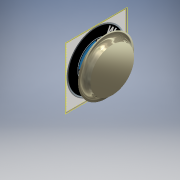
# Autodesk Inventor part: BMW Cap dish decal ready to attach
Saved by Autodesk Inventor 2016 (Build 200138000, 138)
## iProperties
Created: 2016-02-13
Part Number: BMW Cap dish decal ready to attach
Material: Brass, Soft Yellow
Document SubType Name: Modeling
Designer: Amilod
Density: 8.47 g/cm^3
Appearance: Nickel
Mass: 13200.3 g
Surface Area: 11659.4 cm^2
Volume: 4888.99 cm^3
Author: Amilod
Autodesk Inventor part; units mm, degrees
ref_plane "XZ Plane" through (0, 0, 0) normal (0, 1, 0) x (-1, 0, 0)
ref_plane "XY Plane" through (0, 0, 0) normal (0, 0, 1) x (1, 0, 0)
ref_plane "Work Plane5" through (-81, 0, 0) normal (1, 0, 0) x (0, 1, 0)
sketch "Sketch9" plane through (-81, 0, 0) normal (1, 0, 0) x (0, 1, 0)
  circle A0 centre (0, 0) radius 36.225
  dimension "d79" = 72.45
  constraints: 1 centre point, 1 coincident
  measures "d79" diameter of A0
extrude "Extrusion5" add sketch "Sketch9" along normal blind 10 draft -8
sketch "Sketch10" plane through (-81, 0, 0) normal (-1, 0, 0) x (0, 0, 1)
  circle A0 centre (0, 0) radius 43.5874
  constraints: 1 centre point, 1 coincident
extrude "Extrusion6" add sketch "Sketch10" along normal blind 1
fillet "Fillet12" radius 8 1 edges at (-81, -36.225, 0)
draft "FaceDraft1" angle 45 pull direction (-1, 0, 0) faces at (-81.6667, -40.4135, -16.3281) fixed edges at (-82, 0, -43.5874)
sketch "Sketch16" plane through (0, 0, 0) normal (0, 1, 0) x (-1, 0, 0)
  line L0 (82, -43.5874) -> (82, 43.5874) projected
  line L1 (82, -43.5874) -> (83.9506, -32.6257) construction
  line L2 (83.9506, -32.6257) -> (84.4455, -26.8642) construction
  line L3 (84.4455, -26.8642) -> (85.3944, -15.8156) construction
  line L4 (85.3944, -15.8156) -> (85.3944, -9.2357) construction
  line L5 (85.3944, -9.2357) -> (84.8986, -0.5811) construction
  line L6 (84.8986, -0.5811) -> (84.8986, 0) construction
  spline S0 degree 4 poles (82, -43.5874) (83.9506, -32.6257) (84.4455, -26.8642) (85.3944, -15.8156) (85.3944, -9.2357) (84.8986, -0.5811) (84.8986, 0) knots 1 1 1 1 1 2 3 4 4 4 4 4
  line L7 (84.8986, 0) -> (82, 0)
  point P0 (0, 0)
  constraints: 2 end point, 1 midpoint, 1 vertical, 3 other
revolve "Revolution3" add sketch "Sketch16" angle 360 about axis through (-84.8986, 0, 0) along (1, 0, 0)
ref_plane "Work Plane7" through (-96.5, 0, 0) normal (1, 0, 0) x (0, 0, -1)
sketch "Sketch23" plane through (-96.5, 0, 0) normal (1, 0, 0) x (0, 0, -1)
  line L0 (-47.6775, 46.8192) -> (46.7277, 46.8192) construction
  line L1 (46.7277, 46.8192) -> (46.7277, -47.7154) construction
  line L2 (46.7277, -47.7154) -> (-47.6775, -47.7154) construction
  line L3 (-47.6775, -47.7154) -> (-47.6775, 46.8192) construction
  point P0 (0, 0)
  constraints: 2 other
body "Solid3"
